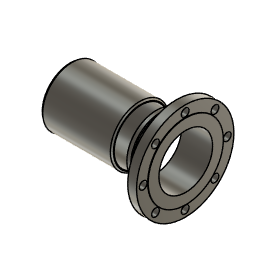
Pipe_Spool_6in (Autodesk Fusion 360 design; units mm, degrees)
part number: 2025-06-04-15-36-36-456
part number: 2025-06-04-15-40-27-177
part number: 2025-06-04-15-43-30-326
Autodesk Fusion 360 part; units mm, degrees
sketch "Sketch1" plane through (0, 0, 0) normal (1, 0, 0) x (0, 1, 0)
  circle A0 centre (0, 0) radius 84.1375
  circle A1 centre (0, 0) radius 77.0255
  dimension "d1" = 168.275
  dimension "d2" = 154.051
  constraint coincident A0.centre A1.centre
  constraint concentric A0 A1
  measures "d1" diameter of A0
  measures "d2" diameter of A1
extrude "Extrude1" add sketch "Sketch1" along normal blind 203.2 makes body 1
copy_body "Body->Comp1" bodies 1 removing the originals makes body 2 in component "Pipe_6_Sch40"
sketch "Sketch1 (2)" plane through (0, 0, 0) normal (1, 0, 0) x (0, 1, 0) in component "Flange_6_150_WN"
  circle A0 centre (0, 0) radius 77.089
  circle A1 centre (0, 0) radius 139.7
  dimension "d5" = 154.178
  dimension "d6" = 279.4
  constraint coincident A0.centre A1.centre
  constraint concentric A0 A1
  measures "d5" diameter of A0
  measures "d6" diameter of A1
extrude "Extrude1'" add sketch "Sketch1 (2)" along normal blind 25.4 separate body makes body 3 in component "Flange_6_150_WN"
sketch "Sketch2" plane through (25.4, 0, 0) normal (1, 0, 0) x (0, 1, 0) in component "Flange_6_150_WN"
  circle A0 centre (0, 0) radius 77.089
  circle A1 centre (0, 0) radius 139.7
  circle A2 centre (0, 0) radius 107.95
  circle A3 centre (0, 0) radius 77.089
  circle A4 centre (0, 0) radius 77.089
  circle A5 centre (0, 0) radius 77.089
  dimension "d9" = 215.9
  constraint concentric A0 A2
  constraint concentric A2 A3
  constraint concentric A2 A4
  constraint concentric A3 A5
  measures "d9" diameter of A2
extrude "Extrude2" add sketch "Sketch2" along normal blind 1.524 contours A2 bodies 3 in component "Flange_6_150_WN"
sketch "Sketch3" plane through (0, 0, 0) normal (-1, 0, 0) x (0, -1, 0) in component "Flange_6_150_WN"
  circle A0 centre (0, 0) radius 77.089
  circle A1 centre (0, 0) radius 139.7
  circle A2 centre (0, 0) radius 96.012
  circle A3 centre (0, 0) radius 77.089
  dimension "d12" = 192.024
  dimension "d13" = 154.178
  constraint concentric A0 A2
  constraint concentric A0 A3
  measures "d12" diameter of A2
  measures "d13" diameter of A3
extrude "Extrude3" add sketch "Sketch3" along normal blind 88.9 separate body contours A2 makes body 4 in component "Flange_6_150_WN"
sketch "Sketch4" plane through (26.924, 0, 0) normal (1, 0, 0) x (0, 1, 0) in component "Flange_6_150_WN"
  circle A0 centre (0, 0) radius 77.089
  circle A1 centre (0, 0) radius 107.95
  circle A2 centre (0, 0) radius 120.65 construction
  circle A3 centre (0, 120.65) radius 11.176
  circle A4 centre (-85.3124, 85.3124) radius 11.176
  circle A5 centre (-120.65, 0) radius 11.176
  circle A6 centre (-85.3124, -85.3124) radius 11.176
  circle A7 centre (0, -120.65) radius 11.176
  circle A8 centre (85.3124, -85.3124) radius 11.176
  circle A9 centre (120.65, 0) radius 11.176
  circle A10 centre (85.3124, 85.3124) radius 11.176
  dimension "d18" = 241.3
  dimension "d19" = 22.352
  dimension "d21" = 360
  constraint coincident A0.centre A1.centre
  constraint coincident A2 A3.centre
  measures "d18" diameter of A2
  measures "d19" diameter of A3
extrude "Extrude4" cut sketch "Sketch4" against normal blind 50.8 contours A3 | A4 | A5 | A6 | A7 | A8 | A9 | A10 bodies 4 3 in component "Flange_6_150_WN"
sketch "Sketch6" plane through (-88.9, 0, 0) normal (-1, 0, 0) x (0, -1, 0) in component "Flange_6_150_WN"
  circle A0 centre (0, 0) radius 77.089
  circle A1 centre (0, 0) radius 96.012
move_body "Move2" bodies 4 to x (1, 0, 0) y (0, 1, 0) z (0, 0, 1) at (26.924, 0, 0) in component "Flange_6_150_WN"
sketch "Sketch7" plane through (-61.976, 0, 0) normal (-1, 0, 0) x (0, -1, 0) in component "Flange_6_150_WN"
  circle A0 centre (0, 0) radius 77.089
  circle A1 centre (0, 0) radius 96.012
  circle A2 centre (0, 0) radius 77.089
  circle A3 centre (0, 0) radius 77.089
  circle A4 centre (0, 0) radius 84.201
  dimension "d30" = 168.402
  constraint coincident A0.centre A1.centre
  constraint concentric A3 A4
  measures "d30" diameter of A4
extrude "Extrude5" cut sketch "Sketch7" against normal blind 15.24 contours A1 bodies 4 in component "Flange_6_150_WN"
chamfer "Chamfer2" distance 66.294 angle 10 1 edges at (-46.736, 89.5146, 34.7194) measured on face at (2.3707, -95.5349, -9.5597) on bodies 4 in component "Flange_6_150_WN"
fillet "Fillet3" radius 80.01 1 edges at (-46.736, 78.6162, 30.4923) on bodies 4 in component "Flange_6_150_WN"
chamfer "Chamfer3" distance 5.08 angle 37.5 1 edges at (-61.976, 78.5029, -30.4484) measured on face at (-61.976, 22.2175, -78.5422) on bodies 4 in component "Flange_6_150_WN"
combine "Combine3" operation add target body 3 tool bodies 4 in component "Flange_6_150_WN"
fillet "Fillet4" radius 6.35 1 edges at (0, 86.2994, 33.4724) on bodies 3 in component "Flange_6_150_WN"
chamfer "Chamfer1" distance 5.08 angle 37.5 2 edges at (203.2, -78.4437, -30.4254) (0, -78.4437, -30.4254) measured on face at (203.2, 81.1668, -8.0067) measured on face at (135.4667, 83.7194, -8.3774) on bodies 2 in component "Pipe_6_Sch40"
draft "Draft4" [suppressed] in component "Flange_6_150_WN"
chamfer "Chamfer1'" [suppressed] in component "Flange_6_150_WN"
combine "Combine2" [suppressed] in component "Flange_6_150_WN"
fillet "Fillet1" [suppressed] in component "Flange_6_150_WN"
move_body "Move1" [suppressed] in component "Flange_6_150_WN"
combine "Combine1" [suppressed] in component "Flange_6_150_WN"
draft "Draft3" [suppressed] in component "Flange_6_150_WN"
component "Pipe_6_Sch40" placed x (1, 0, 0) y (0, 1, 0) z (0, 0, 1) at (0, 0, 0)
component "Flange_6_150_WN" placed x (1, 0, 0) y (0, 1, 0) z (0, 0, 1) at (0, 0, 1.3462)
named bodies: "Pipe_6_Sch40", "Flange"
